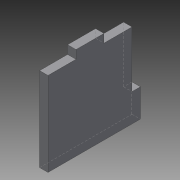
# Autodesk Inventor part: Motor Side support
Saved by Autodesk Inventor 2015 (Build 190159000, 159)
## iProperties
Created: 2014-07-27
Part Number: Motor Side support
Material: Generic
Document SubType Name: Modeling
Designer: karl
Density: 1 g/cm^3
Appearance: Default
Author: karl
Autodesk Inventor part; units mm, degrees
ref_plane "YZ Plane" through (0, 0, 0) normal (1, 0, 0) x (0, 1, 0)
ref_plane "XZ Plane" through (0, 0, 0) normal (0, 1, 0) x (-1, 0, 0)
ref_plane "XY Plane" through (0, 0, 0) normal (0, 0, 1) x (1, 0, 0)
sketch "Sketch1" plane through (0, 0, 0) normal (1, 0, 0) x (0, 1, 0)
  line L0 (15, -15) -> (-15, -15)
  line L1 (-15, -15) -> (-15, 15)
  line L2 (-15, 15) -> (15, 15)
  line L3 (15, 15) -> (15, -15)
  line L4 (15, -15) -> (-15, 15) construction
  line L5 (-15, -15) -> (15, 15) construction
  line L6 (15, -15) -> (18, -15)
  line L7 (18, -15) -> (18, -5)
  line L8 (18, -5) -> (15, -5)
  line L9 (15, -5) -> (15, -15)
  line L10 (-5, 15) -> (5, 15)
  line L11 (5, 15) -> (5, 18)
  line L12 (5, 18) -> (-5, 18)
  line L13 (-5, 18) -> (-5, 15)
  point P0 (0, 0)
  point P1 (0, 18)
  point P2 (0, 0)
  dimension "d0" = 30
  dimension "d1" = 30
  dimension "d2" = 3
  dimension "d3" = 10
  dimension "d4" = 10
  dimension "d5" = 3
  constraints: 28 end point, 6 parallel, 4 midpoint, 3 horizontal, 3 perpendicular, 1 point on line, 1 vertical alignment
  measures "d0" distance of L1.end L2.end
  measures "d1" distance of L0.end L1.end
  measures "d2" distance of L8.end L7.end
  measures "d3" distance of L7.end L6.end
  measures "d4" distance of L12.end L11.end
  measures "d5" distance of L11.end L10.end
extrude "Extrusion1" add sketch "Sketch1" along normal blind 3
sketch "Sketch2" plane through (0, 0, 0) normal (-1, 0, 0) x (0, 0, 1)
  line L0 (15, -15) -> (-15, -15) projected
  line L1 (-15, -15) -> (-15, 18) projected
  line L2 (10, 10) -> (-10, 10)
  line L3 (-10, 10) -> (-10, -10)
  line L4 (-10, -10) -> (10, -10)
  line L5 (10, -10) -> (10, 10)
  line L6 (10, 10) -> (-10, -10) construction
  line L7 (-10, 10) -> (10, -10) construction
  point P0 (0, 0)
  dimension "d8" = 5
  dimension "d9" = 5
  constraints: 12 end point, 2 midpoint, 2 parallel, 1 horizontal, 1 perpendicular
  measures "d8" distance between parallel lines of L0 L4
  measures "d9" distance between parallel lines of L1 L3
extrude "Extrusion2" cut sketch "Sketch2" against normal blind 3
sketch "Sketch3" plane through (0, 0, 0) normal (-1, 0, 0) x (0, 0, 1)
  line L0 (10, -10) -> (-10, -10) projected
  line L1 (10, 10) -> (10, -10) projected
  line L2 (-8.9393, 11.0607) -> (11.0607, -8.9393)
  line L3 (11.0607, -8.9393) -> (8.9393, -11.0607)
  line L4 (8.9393, -11.0607) -> (-11.0607, 8.9393)
  line L5 (-11.0607, 8.9393) -> (-8.9393, 11.0607)
  line L6 (-8.9393, 11.0607) -> (8.9393, -11.0607) construction
  line L7 (11.0607, -8.9393) -> (-11.0607, 8.9393) construction
  point P0 (0, 0)
  dimension "d12" = 3
  constraints: 12 end point, 2 midpoint, 2 parallel, 1 perpendicular
  measures "d12" distance of L2.end L3.end
extrude "Extrusion3" add sketch "Sketch3" against normal blind 3
equation "\"d9\" = d8"
body "Solid1"
